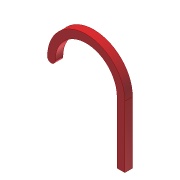
# Autodesk Inventor part: HangHook
Saved by Autodesk Inventor 2012 (Build 160160000, 160)
## iProperties
Created: 2013-01-22
Part Number: HangHook
Material: Steel, High Strength Low Alloy
Document SubType Name: Modeling
Designer: JesseK
Density: 7.84 g/cm^3
Mass: 45.2157 g
Surface Area: 37.0494 cm^2
Volume: 5.76731 cm^3
Author: JesseK
Autodesk Inventor part; units mm, degrees
ref_plane "YZ Plane" through (0, 0, 0) normal (1, 0, 0) x (0, 1, 0)
ref_plane "XZ Plane" through (0, 0, 0) normal (0, 1, 0) x (-1, 0, 0)
ref_plane "XY Plane" through (0, 0, 0) normal (0, 0, 1) x (1, 0, 0)
sketch "Sketch1" plane through (0, 0, 0) normal (0, 0, 1) x (1, 0, 0)
  arc A0 (25.4, 0) -> (-25.4, 0.0312) centre (0, 0) ccw
  arc A1 (31.75, 0) -> (-31.75, 0.039) centre (0, 0) ccw
  arc A2 (-31.75, 0.039) -> (-25.4, 0.0312) centre (-28.575, 0.0351) ccw
  line L0 (25.4, 0) -> (25.4, -50.8)
  line L1 (25.4, -50.8) -> (31.75, -50.8)
  line L2 (31.75, -50.8) -> (31.75, 0)
  line L3 (25.4, 0) -> (31.75, 0) construction
  dimension "d0" = 6.35
  dimension "d1" = 25.4
  dimension "d2" = 50.8
  constraints: 8 end point, 6 point on circle, 3 centre point, 3 tangent, 2 coincident, 2 horizontal, 2 vertical
  measures "d0" distance of L0.end L1.end
  measures "d1" radius of A0
  measures "d2" distance of L1.end L2.end
extrude "Extrusion1" add sketch "Sketch1" along normal blind 6.35
body "Solid1"
